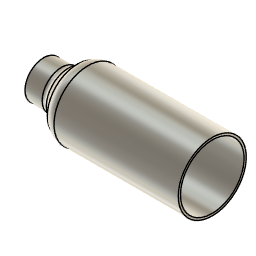
bandsaw_dust_extracion_adapter (Autodesk Fusion 360 design; units mm, degrees)
Autodesk Fusion 360 part; units mm, degrees
sketch "Sketch1" plane through (0, 0, 0) normal (0, 1, 0) x (1, 0, 0)
  line L0 (0, 0) -> (0, -20)
  line L1 (0, 0) -> (155, 0)
  line L2 (155, 0) -> (155, 20)
  line L3 (155, 20) -> (182.5, 20)
  line L4 (182.5, 20) -> (182.5, 36)
  line L5 (182.5, 36) -> (204.5, 36)
  line L6 (204.5, 36) -> (204.5, 41)
  line L7 (204.5, 41) -> (104.5, 41)
  dimension "d1" = 20
  dimension "d2" = 155
  dimension "d11" = 20
  dimension "d12" = 27.5
  dimension "d13" = 16
  dimension "d14" = 22
  dimension "d15" = 5
  dimension "d16" = 100
  constraint coincident L0.start L1.start
  constraint vertical L0
  constraint perpendicular L0 L1
  constraint perpendicular L1 L2
  constraint perpendicular L2 L3
  constraint perpendicular L3 L4
  constraint perpendicular L4 L5
  constraint perpendicular L5 L6
  constraint perpendicular L6 L7
  measures "d1" distance of L0.start L0.end
  measures "d2" distance of L0.start L1.end
  measures "d11" distance of L1.end L2.end
  measures "d12" distance of L2.end L3.end
  measures "d13" distance of L3.end L4.end
  measures "d14" distance of L4.end L5.end
  measures "d15" distance of L5.end L6.end
  measures "d16" distance of L6.end L7.end
sketch "Sketch2" plane through (0, 0, 0) normal (1, 0, 0) x (0, 1, 0)
  line L0 (0, 0) -> (0, 20)
  line L1 (0, 20) -> (0, 37.25) construction
  circle A0 centre (0, 37.25) radius 17.25
  circle A1 centre (0, 37.25) radius 15.75
  point P0 (0, 20)
  dimension "d3" = 17.25
  dimension "d4" = -1.5
  constraint coincident P0 L0.end
  constraint parallel L0 L1
  constraint coincident L1.end A0.centre
  constraint coincident P0 A0
  measures "d3" distance of P0 L1.end
ref_plane "WorkPlane1" through (20, 0, 0) normal (1, 0, 0) x (0, 1, 0)
sketch "Sketch3" plane through (20, 0, 0) normal (1, 0, 0) x (0, 1, 0)
  circle A0 centre (0, 37.25) radius 15.75 construction
  circle A1 centre (0, 37.25) radius 17.9
  circle A2 centre (0, 37.25) radius 16.4
  dimension "d6" = 35.8
  dimension "d7" = -1.5
  constraint concentric A0 A1
  measures "d6" diameter of A1
loft "Loft1" add profiles "Sketch2", "Sketch3" section 1 section 2
loft "Loft2" cut profiles "Sketch3", "Sketch2" section 1 contours A2 section 2 contours A1
ref_plane "WorkPlane2" through (35, 0, 37.25) normal (1, 0, 0) x (0, 1, 0)
sketch "Sketch4" plane through (35, 0, 0) normal (1, 0, 0) x (0, 1, 0)
  circle A0 centre (0, 37.25) radius 16.4 construction
  circle A1 centre (0, 37.25) radius 29.25
  circle A2 centre (0, 37.25) radius 31.25
  dimension "d9" = 58.5
  dimension "d10" = 2
  constraint concentric A0 A1
  measures "d9" diameter of A1
loft "Loft3" add profiles "Sketch3", "Sketch4" section 1 contours A1 | A2 section 2 contours A1 | A2
loft "Loft4" cut profiles "Sketch4", "Sketch3" section 1 contours A1 section 2 contours A2
extrude "Extrude1" add sketch "Sketch4" along normal blind 120
fillet "Fillet1" radius 10 2 edges at (20, -15.2902, 43.1805) (20, -16.6887, 43.7229)
fillet "Fillet2" radius 15 2 edges at (35, -27.2706, 47.8273) (35, -29.1352, 48.5505)
equation "d3 = ( 34.5 / 2 ) * 1 mm"
